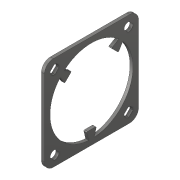
# Autodesk Inventor part: Harting Gasket 1
Saved by Autodesk Inventor 2019.3 (Build 233278000, 278)
## iProperties
Created: 2019-03-15
Part Number: Harting Gasket 1
Material: Generic
Document SubType Name: Modeling
Designer: Kathryn Rosie
Density: 1 g/cm^3
Appearance: Rubber - Black - Version 1.1
Author: Kathryn Rosie
Autodesk Inventor part; units mm, degrees
ref_plane "YZ Plane" through (0, 0, 0) normal (1, 0, 0) x (0, 1, 0)
ref_plane "XZ Plane" through (0, 0, 0) normal (0, 1, 0) x (-1, 0, 0)
ref_plane "XY Plane" through (0, 0, 0) normal (0, 0, 1) x (1, 0, 0)
sketch "Sketch1" plane through (0, 0, 0) normal (1, 0, 0) x (0, 1, 0)
  line L0 (-12.75, 15.75) -> (12.75, 15.75)
  line L1 (15.75, 12.75) -> (15.75, -12.75)
  line L2 (12.75, -15.75) -> (-12.75, -15.75)
  line L3 (-15.75, -12.75) -> (-15.75, 12.75)
  line L4 (-15.75, 15.75) -> (15.75, -15.75) construction
  line L5 (15.75, 15.75) -> (-15.75, -15.75) construction
  line L6 (15.75, 15.75) -> (-15.75, -15.75)
  line L7 (7.9011, 23.5989) -> (-23.5989, -7.9011)
  circle A0 centre (0, 0) radius 17.5 construction
  line L8 (28.1244, 3.3756) -> (-3.3756, -28.1244) construction
  arc A1 (10.8821, -12.2221) -> (11.3137, -13.435) centre (12.3744, -12.3744) ccw
  arc A2 (13.435, -11.3137) -> (12.2221, -10.8821) centre (12.3744, -12.3744) ccw
  arc A3 (10.8821, -12.2221) -> (12.2221, -10.8821) centre (0, 0) ccw
  arc A4 (11.3137, -13.435) -> (12.5266, -13.8666) centre (12.3744, -12.3744) ccw
  arc A5 (13.8666, -12.5266) -> (13.435, -11.3137) centre (12.3744, -12.3744) ccw
  arc A6 (13.8666, -12.5266) -> (12.5266, -13.8666) centre (24.7487, -24.7487) ccw
  arc A7 (12.5266, 13.8666) -> (11.3137, 13.435) centre (12.3744, 12.3744) ccw
  arc A8 (12.5266, 13.8666) -> (13.8666, 12.5266) centre (24.7487, 24.7487) ccw
  arc A9 (13.435, 11.3137) -> (13.8666, 12.5266) centre (12.3744, 12.3744) ccw
  arc A10 (12.2221, 10.8821) -> (13.435, 11.3137) centre (12.3744, 12.3744) ccw
  arc A11 (12.2221, 10.8821) -> (10.8821, 12.2221) centre (0, 0) ccw
  arc A12 (11.3137, 13.435) -> (10.8821, 12.2221) centre (12.3744, 12.3744) ccw
  arc A13 (-13.8666, 12.5266) -> (-13.435, 11.3137) centre (-12.3744, 12.3744) ccw
  arc A14 (-13.8666, 12.5266) -> (-12.5266, 13.8666) centre (-24.7487, 24.7487) ccw
  arc A15 (-11.3137, 13.435) -> (-12.5266, 13.8666) centre (-12.3744, 12.3744) ccw
  arc A16 (-10.8821, 12.2221) -> (-11.3137, 13.435) centre (-12.3744, 12.3744) ccw
  arc A17 (-10.8821, 12.2221) -> (-12.2221, 10.8821) centre (0, 0) ccw
  arc A18 (-13.435, 11.3137) -> (-12.2221, 10.8821) centre (-12.3744, 12.3744) ccw
  arc A19 (-12.5266, -13.8666) -> (-11.3137, -13.435) centre (-12.3744, -12.3744) ccw
  arc A20 (-12.5266, -13.8666) -> (-13.8666, -12.5266) centre (-24.7487, -24.7487) ccw
  arc A21 (-13.435, -11.3137) -> (-13.8666, -12.5266) centre (-12.3744, -12.3744) ccw
  arc A22 (-12.2221, -10.8821) -> (-13.435, -11.3137) centre (-12.3744, -12.3744) ccw
  arc A23 (-12.2221, -10.8821) -> (-10.8821, -12.2221) centre (0, 0) ccw
  arc A24 (-11.3137, -13.435) -> (-10.8821, -12.2221) centre (-12.3744, -12.3744) ccw
  arc A25 (15.75, 12.75) -> (12.75, 15.75) centre (12.75, 12.75) ccw
  arc A26 (-12.75, 15.75) -> (-15.75, 12.75) centre (-12.75, 12.75) ccw
  arc A27 (-15.75, -12.75) -> (-12.75, -15.75) centre (-12.75, -12.75) ccw
  arc A28 (12.75, -15.75) -> (15.75, -12.75) centre (12.75, -12.75) ccw
  line L9 (9.1716, -6.9652) -> (10.4759, -9.1359)
  line L10 (-15.0803, 16.4203) -> (16.4197, -15.0797) construction
  line L11 (6.9652, -9.1716) -> (9.1359, -10.4759)
  line L12 (-16.4203, 15.0803) -> (15.0797, -16.4197) construction
  line L13 (23.5989, 7.9011) -> (15.75, 0.0522)
  line L14 (8.7806, -6.9172) -> (6.9172, -8.7806)
  arc A29 (9.1716, -6.9652) -> (8.7806, -6.9172) centre (8.9573, -7.094) ccw
  arc A30 (6.9172, -8.7806) -> (6.9652, -9.1716) centre (7.094, -8.9573) ccw
  line L15 (9.1716, 6.9652) -> (10.4759, 9.1359)
  arc A31 (8.7806, 6.9172) -> (9.1716, 6.9652) centre (8.9573, 7.094) ccw
  line L16 (6.9172, 8.7806) -> (8.7806, 6.9172)
  arc A32 (6.9652, 9.1716) -> (6.9172, 8.7806) centre (7.094, 8.9573) ccw
  line L17 (6.9652, 9.1716) -> (9.1359, 10.4759)
  line L18 (-11.4105, 1.5602) -> (-13.8677, 0.9475)
  arc A33 (-11.1, 1.3176) -> (-11.4105, 1.5602) centre (-11.35, 1.3176) ccw
  arc A34 (-11.4105, -1.5602) -> (-11.1, -1.3176) centre (-11.35, -1.3176) ccw
  line L19 (-11.1, -1.3176) -> (-11.1, 1.3176)
  line L20 (-11.4105, -1.5602) -> (-13.8677, -0.9475)
  arc A35 (10.4759, -9.1359) -> (10.4759, 9.1359) centre (0, 0) ccw
  arc A36 (9.1359, 10.4759) -> (-13.8677, 0.9475) centre (0, 0) ccw
  arc A37 (-13.8677, -0.9475) -> (9.1359, -10.4759) centre (0, 0) ccw
  point P0 (9.0068, -6.691)
  point P1 (6.691, -9.0068)
  point P2 (9.0068, 6.691)
  point P3 (6.691, 9.0068)
  point P4 (-11.1, 1.6376)
  point P5 (-11.1, -1.6376)
  dimension "d10" = 35
  dimension "d0" = 31.5
  dimension "d1" = 31.5
  dimension "d4" = 11.1
  dimension "d17" = 360
  dimension "d19" = 3
  dimension "d21" = 0.25
  dimension "d22" = 0.25
  dimension "d25" = 90
  dimension "d29" = 135
  constraints: 74 point on circle, 42 end point, 37 centre point, 27 point on line, 12 tangent, 7 symmetric about line, 6 parallel, 3 coincident, 3 equal radius, 2 midpoint, 1 horizontal, 1 perpendicular, 99 other
  measures "d0" distance of L4.end L5.end
  measures "d1" distance of L5.start L4.end
  measures "d4" distance between parallel lines of L5 L7
  measures "d19" radius of A25
  measures "d21" radius of A29
  measures "d22" radius of A30
extrude "Extrusion1" add sketch "Sketch1" along normal blind 1 contours L0 L7 A36 L3 A26 | L0 A25 L6 A8 A7 A12 A11 L16 A32 L17 A36 L7 | L7 A36 L18 A33 L19 A34 L20 A37 L6 A23 A22 A21 A20 A27 L3 | A25 L1 A28 L2 A27 L6 A20 A19 A24 A23 A37 L11 A30 L14 A29 L9 A35 L15 A31 L16 A11 A10 A9 A8
body "Solid1"
